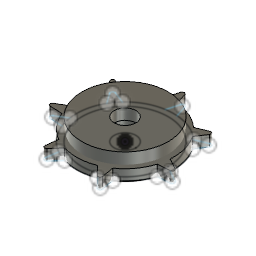
sprocket_9mm (Autodesk Fusion 360 design; units mm, degrees)
Autodesk Fusion 360 part; units mm, degrees
sketch "スケッチ1" plane through (0, 0, 0) normal (0, 0, 1) x (1, 0, 0)
  circle A0 centre (0, 0) radius 4.5
  line L0 (-0.3926, 5.5537) -> (-0.7019, 4.4449)
  line L1 (0.3344, 4.4876) -> (-0.0095, 5.561)
  arc A1 (-0.0095, 5.561) -> (-0.3926, 5.5537) centre (-0.2, 5.5) ccw
  arc A2 (-4.3537, 3.4598) -> (-4.5869, 3.1557) centre (-4.4248, 3.2728) ccw
  line L2 (-4.5869, 3.1557) -> (-3.9128, 2.2226)
  line L3 (-3.3, 3.0594) -> (-4.3537, 3.4598)
  arc A3 (-5.4195, -1.2467) -> (-5.3271, -1.6186) centre (-5.3176, -1.4189) ccw
  line L4 (-5.3271, -1.6186) -> (-4.1773, -1.6734)
  line L5 (-4.4494, -0.6726) -> (-5.4195, -1.2467)
  arc A4 (-2.4042, -5.0144) -> (-2.0559, -5.1741) centre (-2.2062, -5.0421) ccw
  line L6 (-2.0559, -5.1741) -> (-1.2962, -4.3093)
  line L7 (-2.2483, -3.8981) -> (-2.4042, -5.0144)
  arc A5 (2.4214, -5.0062) -> (2.7634, -4.8334) centre (2.5666, -4.8686) ccw
  line L8 (2.7634, -4.8334) -> (2.5609, -3.7002)
  line L9 (1.6458, -4.1882) -> (2.4214, -5.0062)
  arc A6 (5.4237, -1.2281) -> (5.5019, -0.853) centre (5.4066, -1.0289) ccw
  line L10 (5.5019, -0.853) -> (4.4897, -0.3048)
  line L11 (4.3006, -1.3245) -> (5.4237, -1.2281)
  arc A7 (4.3418, 3.4747) -> (4.0973, 3.7697) centre (4.1754, 3.5856) ccw
  line L12 (4.0973, 3.7697) -> (3.0376, 3.3201)
  line L13 (3.717, 2.5365) -> (4.3418, 3.4747)
  circle A8 centre (0, 0) radius 1
  circle A9 centre (0, 0) radius 4
  dimension "d1" = 9
  dimension "d2" = 0.2
  dimension "d4" = 360
  dimension "d5" = 2
  dimension "d10" = 8
  constraint coincident A0.centre A8.centre
  constraint coincident A0 L0.end
  constraint coincident A0 L1.start
  constraint tangent L0 A1
  constraint tangent L1 A1
  constraint concentric A0 A8
  measures "d1" diameter of A0
  measures "d2" radius of A1
  measures "d5" diameter of A8
  measures "d10" diameter of A9
extrude "押し出し1" add sketch "スケッチ1" along normal blind 1 contours A0 | A0 A7 L12 L13 | A0 A6 L10 L11 | A0 L0 L1 A1 | A0 A5 L8 L9 | A0 A2 L2 L3 | A0 A4 L6 L7 | A0 A3 L4 L5 | A8 | A9 makes body 1
extrude "押し出し2" cut sketch "スケッチ1" along normal blind 1 contours A8 bodies 1
extrude "押し出し3" add sketch "スケッチ1" along normal blind 2 and the other way blind 0 separate body contours A9 makes body 2
